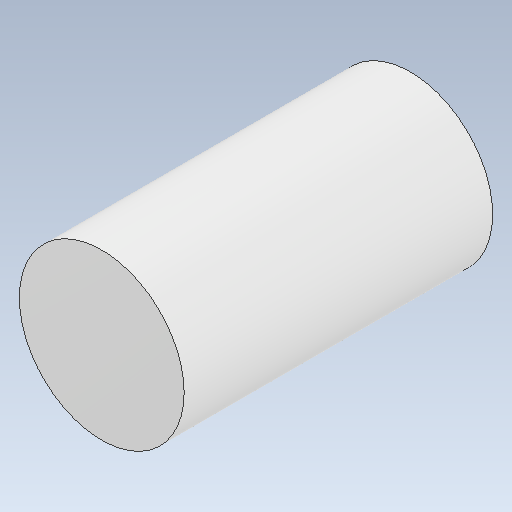
# Autodesk Inventor part: 8011_1uF_Tx_Capacitor_v1
Saved by Autodesk Inventor 2021 (Build 250183000, 183)
## iProperties
Created: 2021-03-01
Part Number: 8011_1uF_Tx_Capacitor_v1
Material: Acetal Resin, White
Document SubType Name: Modeling
Designer: Barksdale
Density: 1.425 g/cm^3
Appearance: Smooth - White
Author: Barksdale
Autodesk Inventor part; units mm, degrees
ref_plane "YZ Plane" through (0, 0, 0) normal (1, 0, 0) x (0, 1, 0)
ref_plane "XZ Plane" through (0, 0, 0) normal (0, 1, 0) x (-1, 0, 0)
ref_plane "XY Plane" through (0, 0, 0) normal (0, 0, 1) x (1, 0, 0)
sketch "Sketch1" plane through (0, 0, 0) normal (0, 0, 1) x (1, 0, 0)
  circle A0 centre (0, 0) radius 11.75
  dimension "d0" = 23.5
  constraints: 1 centre point, 1 coincident
  measures "d0" diameter of A0
extrude "Extrusion1" add sketch "Sketch1" along normal blind 44
body "Solid1"
